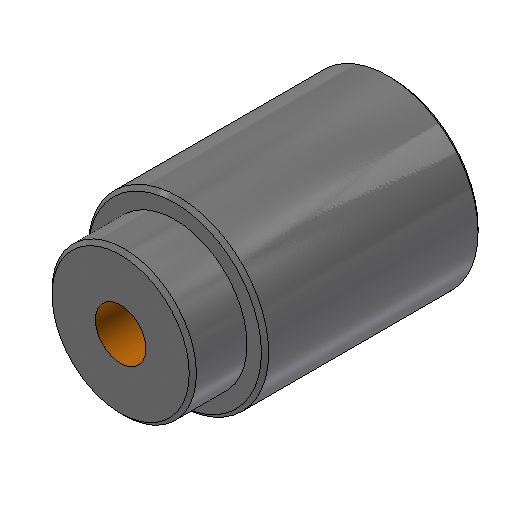
# Autodesk Inventor part: TL20240701-10110CV-020
Saved by Autodesk Inventor 2022.5 (Build 265521000, 521)
## iProperties
Category: DRIVE UNIT ASSY
Manager: 호상태
Company: 현대 트랜시스(대유)
RuleStatus: InUse
Created: 2023-01-19
Part Number: TL20240701-10110CV-020
Project: SW PJT
Checked By: 김형민
Engr Approved By: 김시현
User Status: 1 x18
Material: S45C
Description: 0
Document SubType Name: Modeling
Mfg Approved By: 호상태
Designer: 박성규
Stock Number: 020
Density: 7.87 g/cm^3
Appearance: Plating Zinc White
BeforeDocSave0: file://Part Design STD iLogic
DETAIL: Coveryor Assembly
M/C TITLE: MEa/NEa차종 시트조립라인
SPECIFICATION: TL20221201-000000CV-004
DocNumber: 221118_Standard_v1
Folder: .\
VDS_Category: 엔지니어링
Detail Description: Processed products
Title: BAR
Subject: SW차종 시트조립라인
Author: 박성규
Revision Number: A
Autodesk Inventor part; units mm, degrees
ref_plane "YZ Plane" through (0, 0, 0) normal (1, 0, 0) x (0, 1, 0)
ref_plane "XZ Plane" through (0, 0, 0) normal (0, 1, 0) x (-1, 0, 0)
ref_plane "XY Plane" through (0, 0, 0) normal (0, 0, 1) x (1, 0, 0)
sketch "스케치8" plane through (0, 0, 0) normal (0, 0, 1) x (1, 0, 0)
  circle A0 centre (0, 0) radius 25
  dimension "d38" = 50
  constraints: 1 centre point, 1 coincident
  measures "d38" diameter of A0
extrude "돌출3" add sketch "스케치8" along normal blind 60
sketch "스케치9" plane through (0, 0, 60) normal (0, 0, 1) x (1, 0, 0)
  circle A0 centre (0, 0) radius 25 construction
  circle A1 centre (0, 0) radius 20
  dimension "d41" = 40
  constraints: 1 centre point, 1 coincident
  measures "d41" diameter of A1
extrude "돌출4" add sketch "스케치9" along normal blind 15
sketch "스케치10" plane through (0, 0, 75) normal (0, 0, 1) x (1, 0, 0)
  circle A0 centre (0, 0) radius 20 construction
  constraints: 1 coincident
hole "구멍3" at (0, 0, 75) direction (0, 0, -1) diameter 14 end through all clearance for "Socket Head Cap Screw" size "M12" standard "TS Profile"
chamfer "모따기1" distance 1 angle 45 3 edges at (-25, 0, 60) (-20, 0, 75) (-25, 0, 0)
